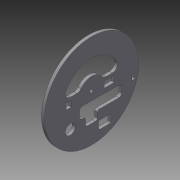
# Autodesk Inventor part: 2.8chassis side DB25V3
Saved by Autodesk Inventor 2015 (Build 190159000, 159)
## iProperties
Created: 2014-05-11
Part Number: 2.8chassis side DB25V3
Material: Generic
Document SubType Name: Modeling
Designer: STACKPOLE
Density: 1 g/cm^3
Appearance: Default
Author: STACKPOLE
Autodesk Inventor part; units mm, degrees
ref_plane "YZ Plane" through (0, 0, 0) normal (1, 0, 0) x (0, 1, 0)
ref_plane "XZ Plane" through (0, 0, 0) normal (0, 1, 0) x (-1, 0, 0)
ref_plane "XY Plane" through (0, 0, 0) normal (0, 0, 1) x (1, 0, 0)
sketch "Sketch1" plane through (0, 0, 0) normal (1, 0, 0) x (0, 1, 0)
  arc A0 (25.215, 12.1739) -> (-25.215, 12.1739) centre (0, 0) ccw
  arc A1 (10.2581, 7.1429) -> (-10.2581, 7.1429) centre (0, 0) ccw
  circle A2 centre (0, 0) radius 1.5
  line L0 (-14.3614, 5) -> (-20.7123, 5)
  line L1 (14.3614, 5) -> (20.7123, 5)
  arc A3 (-25.215, 12.1739) -> (-20.7123, 5) centre (-20.7123, 10) ccw
  arc A4 (-14.3614, 5) -> (-10.2581, 7.1429) centre (-14.3614, 10) ccw
  arc A5 (10.2581, 7.1429) -> (14.3614, 5) centre (14.3614, 10) ccw
  arc A6 (20.7123, 5) -> (25.215, 12.1739) centre (20.7123, 10) ccw
  line L2 (27, -8.5) -> (-9, -8.5)
  line L3 (-12, -11.5) -> (-12, -8.988)
  arc A7 (-9, -8.5) -> (-12, -11.5) centre (-9, -11.5) ccw
  line L4 (-9, -19.5) -> (27, -19.5)
  line L5 (30, -16.5) -> (30, -11.5)
  circle A8 centre (0, 0) radius 46.5
  line L6 (-12, -11.5) -> (-12, -16.5)
  arc A9 (-12, -16.5) -> (-9, -19.5) centre (-9, -16.5) ccw
  arc A10 (27, -19.5) -> (30, -16.5) centre (27, -16.5) ccw
  arc A11 (30, -11.5) -> (27, -8.5) centre (27, -11.5) ccw
  point P0 (7.4416, -10.0435)
  point P1 (-11.4564, 5)
  point P2 (11.4564, 5)
  point P3 (-27.55, 5)
  point P4 (27.55, 5)
  dimension "d5" = 28
  dimension "d6" = 25
  dimension "d7" = 3
  dimension "d53" = 5
  dimension "d54" = 5
  dimension "d86" = 12
  dimension "d90" = 8.5
  dimension "d91" = 3
  dimension "d95" = 93
  dimension "d96" = 3
  dimension "d97" = 42
  dimension "d98" = 11
  constraints: 25 point on circle, 16 tangent, 14 end point, 12 centre point, 5 equal radius, 4 coincident, 4 point on line, 3 horizontal, 2 collinear, 2 perpendicular, 1 vertical
  measures "d5" radius of A0
  measures "d6" diameter of A1
  measures "d7" diameter of A2
  measures "d53" distance from line of point (0, 0) L1
  measures "d54" radius of A3
  measures "d86" horizontal distance of L3.end point (0, 0)
  measures "d90" distance from line of point (0, 0) L2
  measures "d91" radius of A7
  measures "d95" diameter of A8
  measures "d96" radius of A9
  measures "d97" distance between parallel lines of L6 L5
  measures "d98" distance between parallel lines of L2 L4
extrude "Extrusion3" add sketch "Sketch1" along normal blind 3
sketch "Sketch2" plane through (3, 0, 0) normal (1, 0, 0) x (0, 0, -1)
  arc A0 (-12.1739, 25.215) -> (-12.1739, -25.215) centre (0, 0) ccw projected
  line L0 (11, 43) -> (6, 43)
  line L1 (6, 43) -> (6, 40)
  line L2 (6, 40) -> (11, 40)
  line L3 (11, 40) -> (11, 43)
  dimension "d99" = 5
  dimension "d100" = 3
  dimension "d101" = 40
  dimension "d102" = 6
  constraints: 8 end point, 2 parallel, 1 horizontal, 1 perpendicular
  measures "d99" distance of L2.end L1.end
  measures "d100" distance of L1.end L0.end
  measures "d101" distance from line of A0.centre L2
  measures "d102" distance from line of L1 A0.centre
extrude "Extrusion5" cut sketch "Sketch2" against normal through all
sketch "Sketch4" plane through (3, 0, 0) normal (1, 0, 0) x (0, 0, -1)
  arc A0 (-12.1739, 25.215) -> (-12.1739, -25.215) centre (0, 0) ccw projected
  line L0 (-2, -20) -> (4, -20)
  line L1 (4, -20) -> (4, -25)
  line L2 (4, -25) -> (-2, -25)
  line L3 (-2, 22.5) -> (4, 22.5)
  line L4 (4, 22.5) -> (4, 12.5)
  line L5 (4, 12.5) -> (-2, 12.5)
  line L6 (-2, 22.5) -> (-2, 12.5)
  line L7 (-5, 20.7123) -> (-5, 14.3614) projected
  line L8 (-2, -20) -> (-2, -25)
  line L9 (6, 40) -> (6, 43) projected
  dimension "d59" = 5
  dimension "d60" = 20
  dimension "d62" = 10
  dimension "d63" = 12.5
  dimension "d94" = 6
  dimension "d104" = 2
  constraints: 16 end point, 2 collinear, 2 horizontal, 2 parallel, 2 perpendicular, 2 vertical
  measures "d59" distance of L0.end L1.end
  measures "d60" distance from line of A0.centre L0
  measures "d62" distance of L3.end L4.end
  measures "d63" distance from line of A0.centre L5
  measures "d94" distance between parallel lines of L6 L4
  measures "d104" distance between parallel lines of L9 L4
extrude "Extrusion6" cut sketch "Sketch4" against normal through all
sketch "Sketch7" plane through (3, 0, 0) normal (1, 0, 0) x (0, 0, -1)
  line L0 (19.5, -6) -> (28, -6)
  line L1 (28, -6) -> (28, 6)
  line L2 (28, 6) -> (19.5, 6)
  line L3 (19.5, 6) -> (19.5, -6)
  line L4 (19.5, 27) -> (19.5, -9) projected
  point P0 (0, 0)
  point P1 (19.5, 0)
  dimension "d105" = 12
  dimension "d106" = 8.5
  constraints: 8 end point, 2 parallel, 1 collinear, 1 horizontal, 1 horizontal alignment, 1 midpoint, 1 perpendicular
  measures "d105" distance of L0.end L1.end
  measures "d106" distance of L1.end L2.end
extrude "Extrusion9" cut sketch "Sketch7" against normal through all
fillet "Fillet1" radius 2 4 edges at (1.5, -6, -19.5) (1.5, -6, -28) (1.5, 6, -28) (1.5, 6, -19.5)
sketch "Sketch8" plane through (0, 0, 0) normal (-1, 0, 0) x (0, 0, 1)
  line L0 (-37, 7) -> (-29, 7)
  line L1 (-29, 7) -> (-29, 19)
  line L2 (-29, 19) -> (-37, 19)
  line L3 (-37, 19) -> (-37, 7)
  point P0 (0, 0)
  dimension "d110" = 12
  dimension "d111" = 8
  dimension "d112" = 29
  dimension "d113" = 7
  constraints: 8 end point, 2 parallel, 1 horizontal, 1 perpendicular
  measures "d110" distance of L0.end L1.end
  measures "d111" distance of L1.end L2.end
  measures "d112" horizontal distance of point (0, 0) L0.end
  measures "d113" vertical distance of point (0, 0) L0.end
extrude "Extrusion10" cut sketch "Sketch8" against normal through all
fillet "Fillet2" radius 1 4 edges at (1.5, 7, -29) (1.5, 7, -37) (1.5, 19, -37) (1.5, 19, -29)
sketch "Sketch9" plane through (0, 0, 0) normal (-1, 0, 0) x (0, 0, 1)
  circle A0 centre (-22.5, -21) radius 5
  point P0 (0, 0)
  dimension "d117" = 10
  dimension "d118" = 22.5
  dimension "d119" = 21
  constraints: 1 centre point
  measures "d117" diameter of A0
  measures "d118" horizontal distance of point (0, 0) A0.centre
  measures "d119" vertical distance of point (0, 0) A0.centre
extrude "Extrusion11" cut sketch "Sketch9" against normal through all
body "Solid3"
